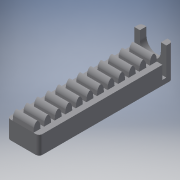
# Autodesk Inventor part: Rack_arms
Saved by Autodesk Inventor 2018 (Build 220112000, 112)
## iProperties
Created: 2017-05-22
Part Number: Rack_arms
Material: Generic
Document SubType Name: Modeling
Designer: nazardio000
Density: 1 g/cm^3
Appearance: Default
Author: nazardio000
Autodesk Inventor part; units mm, degrees
ref_plane "YZ Plane" through (0, 0, 0) normal (1, 0, 0) x (0, 1, 0)
ref_plane "XZ Plane" through (0, 0, 0) normal (0, 1, 0) x (-1, 0, 0)
ref_plane "XY Plane" through (0, 0, 0) normal (0, 0, 1) x (1, 0, 0)
sketch "Sketch2" plane through (0, 0, 0) normal (1, 0, 0) x (0, 1, 0)
  line L0 (-5.5245, 31.75) -> (-5.5245, -31.75)
  line L1 (-5.5245, -31.75) -> (5.5245, -31.75)
  line L2 (5.5245, -31.75) -> (5.5245, 31.75)
  line L3 (5.5245, 31.75) -> (-5.5245, 31.75)
  line L4 (-5.5245, 31.75) -> (5.5245, -31.75) construction
  line L5 (-5.5245, -31.75) -> (5.5245, 31.75) construction
  point P0 (0, 0)
  dimension "d4" = 63.5
  dimension "d5" = 11.049
  constraints: 12 end point, 2 midpoint, 2 parallel, 1 perpendicular, 1 vertical
  measures "d4" distance of L0.start L0.end
  measures "d5" distance of L1.end L0.end
extrude "Extrusion2" add sketch "Sketch2" along normal mid plane 9.779
sketch "Sketch3" plane through (0, 0, 0) normal (1, 0, 0) x (0, 1, 0)
  line L0 (5.5245, -31.75) -> (5.5245, 31.75) projected
  line L1 (5.5245, 31.9532) -> (5.5245, 29.4132)
  line L2 (5.5245, 31.9532) -> (5.5245, 29.4132)
  arc A0 (8.0645, 30.8543) -> (6.7945, 31.629) centre (6.3804, 29.5218) ccw
  line L3 (8.0645, 30.6737) -> (7.6408, 30.6737)
  arc A1 (6.7945, 29.7184) -> (8.0645, 30.4931) centre (6.3804, 31.8256) ccw
  line L4 (8.0645, 30.8543) -> (8.0645, 30.4931)
  line L5 (5.5245, 31.75) -> (5.5245, -31.75)
  arc A2 (8.0642, -1.6042) -> (8.0645, -1.6033) centre (6.6313, -1.0154) ccw
  line L6 (6.7945, 31.629) -> (5.5245, 31.7489)
  line L7 (6.7945, 29.7184) -> (5.5245, 29.5986)
  line L8 (5.5245, 31.7489) -> (6.7945, 31.629)
  line L9 (6.7945, 29.7184) -> (5.5245, 29.5986)
  line L10 (5.5245, 29.5986) -> (5.5245, 31.7489)
  arc A3 (8.0645, 30.8543) -> (6.7945, 31.629) centre (6.3804, 29.5218) ccw
  arc A4 (6.7945, 29.7184) -> (8.0645, 30.4931) centre (6.3804, 31.8256) ccw
  line L11 (8.0645, 30.8543) -> (8.0645, 30.4931)
  line L12 (8.0645, 27.4448) -> (7.6408, 27.4448)
  line L13 (8.0645, 27.6255) -> (8.0645, 27.2642)
  line L14 (8.0645, 27.6255) -> (8.0645, 27.2642)
  arc A5 (6.7945, 26.4895) -> (8.0645, 27.2642) centre (6.3804, 28.5967) ccw
  arc A6 (8.0645, 27.6255) -> (6.7945, 28.4002) centre (6.3804, 26.293) ccw
  arc A7 (6.7945, 26.4895) -> (8.0645, 27.2642) centre (6.3804, 28.5967) ccw
  arc A8 (8.0645, 27.6255) -> (6.7945, 28.4002) centre (6.3804, 26.293) ccw
  line L15 (5.5245, 28.5211) -> (5.5245, -34.9788)
  line L16 (5.5245, 28.7243) -> (5.5245, 26.1843)
  line L17 (6.7945, 26.4895) -> (5.5245, 26.3697)
  line L18 (5.5245, 28.52) -> (6.7945, 28.4002)
  line L19 (6.7945, 26.4895) -> (5.5245, 26.3697)
  line L20 (5.5245, 26.3697) -> (5.5245, 28.52)
  line L21 (5.5245, 28.7243) -> (5.5245, 26.1843)
  line L22 (6.7945, 28.4002) -> (5.5245, 28.52)
  line L23 (8.0645, 24.216) -> (7.6408, 24.216)
  line L24 (8.0645, 24.3966) -> (8.0645, 24.0353)
  line L25 (8.0645, 24.3966) -> (8.0645, 24.0353)
  arc A9 (6.7945, 23.2606) -> (8.0645, 24.0353) centre (6.3804, 25.3678) ccw
  arc A10 (8.0645, 24.3966) -> (6.7945, 25.1713) centre (6.3804, 23.0641) ccw
  arc A11 (6.7945, 23.2606) -> (8.0645, 24.0353) centre (6.3804, 25.3678) ccw
  arc A12 (8.0645, 24.3966) -> (6.7945, 25.1713) centre (6.3804, 23.0641) ccw
  line L26 (5.5245, 25.2923) -> (5.5245, -38.2077)
  line L27 (5.5245, 25.4955) -> (5.5245, 22.9555)
  line L28 (6.7945, 23.2606) -> (5.5245, 23.1408)
  line L29 (5.5245, 25.2911) -> (6.7945, 25.1713)
  line L30 (6.7945, 23.2606) -> (5.5245, 23.1408)
  line L31 (5.5245, 23.1408) -> (5.5245, 25.2911)
  line L32 (5.5245, 25.4955) -> (5.5245, 22.9555)
  line L33 (6.7945, 25.1713) -> (5.5245, 25.2911)
  line L34 (8.0645, 20.9871) -> (7.6408, 20.9871)
  line L35 (8.0645, 21.1677) -> (8.0645, 20.8065)
  line L36 (8.0645, 21.1677) -> (8.0645, 20.8065)
  arc A13 (6.7945, 20.0318) -> (8.0645, 20.8065) centre (6.3804, 22.139) ccw
  arc A14 (8.0645, 21.1677) -> (6.7945, 21.9424) centre (6.3804, 19.8352) ccw
  arc A15 (6.7945, 20.0318) -> (8.0645, 20.8065) centre (6.3804, 22.139) ccw
  arc A16 (8.0645, 21.1677) -> (6.7945, 21.9424) centre (6.3804, 19.8352) ccw
  line L37 (5.5245, 22.0634) -> (5.5245, -41.4366)
  line L38 (5.5245, 22.2666) -> (5.5245, 19.7266)
  line L39 (6.7945, 20.0318) -> (5.5245, 19.9119)
  line L40 (5.5245, 22.0623) -> (6.7945, 21.9424)
  line L41 (6.7945, 20.0318) -> (5.5245, 19.9119)
  line L42 (5.5245, 19.9119) -> (5.5245, 22.0623)
  line L43 (5.5245, 22.2666) -> (5.5245, 19.7266)
  line L44 (6.7945, 21.9424) -> (5.5245, 22.0623)
  line L45 (8.0645, 17.7582) -> (7.6408, 17.7582)
  line L46 (8.0645, 17.9389) -> (8.0645, 17.5776)
  line L47 (8.0645, 17.9389) -> (8.0645, 17.5776)
  arc A17 (6.7945, 16.8029) -> (8.0645, 17.5776) centre (6.3804, 18.9101) ccw
  arc A18 (8.0645, 17.9389) -> (6.7945, 18.7136) centre (6.3804, 16.6064) ccw
  arc A19 (6.7945, 16.8029) -> (8.0645, 17.5776) centre (6.3804, 18.9101) ccw
  arc A20 (8.0645, 17.9389) -> (6.7945, 18.7136) centre (6.3804, 16.6064) ccw
  line L48 (5.5245, 18.8345) -> (5.5245, -44.6655)
  line L49 (5.5245, 19.0377) -> (5.5245, 16.4977)
  line L50 (6.7945, 16.8029) -> (5.5245, 16.6831)
  line L51 (5.5245, 18.8334) -> (6.7945, 18.7136)
  line L52 (6.7945, 16.8029) -> (5.5245, 16.6831)
  line L53 (5.5245, 16.6831) -> (5.5245, 18.8334)
  line L54 (5.5245, 19.0377) -> (5.5245, 16.4977)
  line L55 (6.7945, 18.7136) -> (5.5245, 18.8334)
  line L56 (8.0645, 14.5294) -> (7.6408, 14.5294)
  line L57 (8.0645, 14.71) -> (8.0645, 14.3487)
  line L58 (8.0645, 14.71) -> (8.0645, 14.3487)
  arc A21 (6.7945, 13.574) -> (8.0645, 14.3487) centre (6.3804, 15.6812) ccw
  arc A22 (8.0645, 14.71) -> (6.7945, 15.4847) centre (6.3804, 13.3775) ccw
  arc A23 (6.7945, 13.574) -> (8.0645, 14.3487) centre (6.3804, 15.6812) ccw
  arc A24 (8.0645, 14.71) -> (6.7945, 15.4847) centre (6.3804, 13.3775) ccw
  line L59 (5.5245, 15.6057) -> (5.5245, -47.8943)
  line L60 (5.5245, 15.8089) -> (5.5245, 13.2689)
  line L61 (6.7945, 13.574) -> (5.5245, 13.4542)
  line L62 (5.5245, 15.6045) -> (6.7945, 15.4847)
  line L63 (6.7945, 13.574) -> (5.5245, 13.4542)
  line L64 (5.5245, 13.4542) -> (5.5245, 15.6045)
  line L65 (5.5245, 15.8089) -> (5.5245, 13.2689)
  line L66 (6.7945, 15.4847) -> (5.5245, 15.6045)
  line L67 (8.0645, 11.3005) -> (7.6408, 11.3005)
  line L68 (8.0645, 11.4811) -> (8.0645, 11.1199)
  line L69 (8.0645, 11.4811) -> (8.0645, 11.1199)
  arc A25 (6.7945, 10.3452) -> (8.0645, 11.1199) centre (6.3804, 12.4524) ccw
  arc A26 (8.0645, 11.4811) -> (6.7945, 12.2558) centre (6.3804, 10.1486) ccw
  arc A27 (6.7945, 10.3452) -> (8.0645, 11.1199) centre (6.3804, 12.4524) ccw
  arc A28 (8.0645, 11.4811) -> (6.7945, 12.2558) centre (6.3804, 10.1486) ccw
  line L70 (5.5245, 12.3768) -> (5.5245, -51.1232)
  line L71 (5.5245, 12.58) -> (5.5245, 10.04)
  line L72 (6.7945, 10.3452) -> (5.5245, 10.2253)
  line L73 (5.5245, 12.3756) -> (6.7945, 12.2558)
  line L74 (6.7945, 10.3452) -> (5.5245, 10.2253)
  line L75 (5.5245, 10.2253) -> (5.5245, 12.3756)
  line L76 (5.5245, 12.58) -> (5.5245, 10.04)
  line L77 (6.7945, 12.2558) -> (5.5245, 12.3756)
  line L78 (8.0645, 8.0716) -> (7.6408, 8.0716)
  line L79 (8.0645, 8.2523) -> (8.0645, 7.891)
  line L80 (8.0645, 8.2523) -> (8.0645, 7.891)
  arc A29 (6.7945, 7.1163) -> (8.0645, 7.891) centre (6.3804, 9.2235) ccw
  arc A30 (8.0645, 8.2523) -> (6.7945, 9.027) centre (6.3804, 6.9198) ccw
  arc A31 (6.7945, 7.1163) -> (8.0645, 7.891) centre (6.3804, 9.2235) ccw
  arc A32 (8.0645, 8.2523) -> (6.7945, 9.027) centre (6.3804, 6.9198) ccw
  line L81 (5.5245, 9.1479) -> (5.5245, -54.3521)
  line L82 (5.5245, 9.3511) -> (5.5245, 6.8111)
  line L83 (6.7945, 7.1163) -> (5.5245, 6.9965)
  line L84 (5.5245, 9.1468) -> (6.7945, 9.027)
  line L85 (6.7945, 7.1163) -> (5.5245, 6.9965)
  line L86 (5.5245, 6.9965) -> (5.5245, 9.1468)
  line L87 (5.5245, 9.3511) -> (5.5245, 6.8111)
  line L88 (6.7945, 9.027) -> (5.5245, 9.1468)
  line L89 (8.0645, 4.8428) -> (7.6408, 4.8428)
  line L90 (8.0645, 5.0234) -> (8.0645, 4.6621)
  line L91 (8.0645, 5.0234) -> (8.0645, 4.6621)
  arc A33 (6.7945, 3.8874) -> (8.0645, 4.6621) centre (6.3804, 5.9946) ccw
  arc A34 (8.0645, 5.0234) -> (6.7945, 5.7981) centre (6.3804, 3.6909) ccw
  arc A35 (6.7945, 3.8874) -> (8.0645, 4.6621) centre (6.3804, 5.9946) ccw
  arc A36 (8.0645, 5.0234) -> (6.7945, 5.7981) centre (6.3804, 3.6909) ccw
  line L92 (5.5245, 5.9191) -> (5.5245, -57.5809)
  line L93 (5.5245, 6.1223) -> (5.5245, 3.5823)
  line L94 (6.7945, 3.8874) -> (5.5245, 3.7676)
  line L95 (5.5245, 5.9179) -> (6.7945, 5.7981)
  line L96 (6.7945, 3.8874) -> (5.5245, 3.7676)
  line L97 (5.5245, 3.7676) -> (5.5245, 5.9179)
  line L98 (5.5245, 6.1223) -> (5.5245, 3.5823)
  line L99 (6.7945, 5.7981) -> (5.5245, 5.9179)
  line L100 (8.0645, 1.6139) -> (7.6408, 1.6139)
  line L101 (8.0645, 1.7945) -> (8.0645, 1.4333)
  line L102 (8.0645, 1.7945) -> (8.0645, 1.4333)
  arc A37 (6.7945, 0.6586) -> (8.0645, 1.4333) centre (6.3804, 2.7658) ccw
  arc A38 (8.0645, 1.7945) -> (6.7945, 2.5692) centre (6.3804, 0.462) ccw
  arc A39 (6.7945, 0.6586) -> (8.0645, 1.4333) centre (6.3804, 2.7658) ccw
  arc A40 (8.0645, 1.7945) -> (6.7945, 2.5692) centre (6.3804, 0.462) ccw
  line L103 (5.5245, 2.6902) -> (5.5245, -60.8098)
  line L104 (5.5245, 2.8934) -> (5.5245, 0.3534)
  line L105 (6.7945, 0.6586) -> (5.5245, 0.5387)
  line L106 (5.5245, 2.689) -> (6.7945, 2.5692)
  line L107 (6.7945, 0.6586) -> (5.5245, 0.5387)
  line L108 (5.5245, 0.5387) -> (5.5245, 2.689)
  line L109 (5.5245, 2.8934) -> (5.5245, 0.3534)
  line L110 (6.7945, 2.5692) -> (5.5245, 2.689)
  line L111 (8.0645, -1.615) -> (7.6408, -1.615)
  line L112 (8.0645, -1.4344) -> (8.0645, -1.7956)
  line L113 (8.0645, -1.4344) -> (8.0645, -1.7956)
  arc A41 (6.7945, -2.5703) -> (8.0645, -1.7956) centre (6.3804, -0.4631) ccw
  arc A42 (8.0645, -1.4344) -> (6.7945, -0.6597) centre (6.3804, -2.7668) ccw
  arc A43 (6.7945, -2.5703) -> (8.0645, -1.7956) centre (6.3804, -0.4631) ccw
  arc A44 (8.0645, -1.4344) -> (6.7945, -0.6597) centre (6.3804, -2.7668) ccw
  line L114 (5.5245, -0.5387) -> (5.5245, -64.0387)
  line L115 (5.5245, -0.3355) -> (5.5245, -2.8755)
  line L116 (6.7945, -2.5703) -> (5.5245, -2.6901)
  line L117 (5.5245, -0.5398) -> (6.7945, -0.6597)
  line L118 (6.7945, -2.5703) -> (5.5245, -2.6901)
  line L119 (5.5245, -2.6901) -> (5.5245, -0.5398)
  line L120 (5.5245, -0.3355) -> (5.5245, -2.8755)
  line L121 (6.7945, -0.6597) -> (5.5245, -0.5398)
  line L122 (8.0645, -4.8438) -> (7.6408, -4.8438)
  line L123 (8.0645, -4.6632) -> (8.0645, -5.0245)
  line L124 (8.0645, -4.6632) -> (8.0645, -5.0245)
  arc A45 (6.7945, -5.7992) -> (8.0645, -5.0245) centre (6.3804, -3.692) ccw
  arc A46 (8.0645, -4.6632) -> (6.7945, -3.8885) centre (6.3804, -5.9957) ccw
  arc A47 (6.7945, -5.7992) -> (8.0645, -5.0245) centre (6.3804, -3.692) ccw
  arc A48 (8.0645, -4.6632) -> (6.7945, -3.8885) centre (6.3804, -5.9957) ccw
  line L125 (5.5245, -3.7676) -> (5.5245, -67.2675)
  line L126 (5.5245, -3.5644) -> (5.5245, -6.1044)
  line L127 (6.7945, -5.7992) -> (5.5245, -5.919)
  line L128 (5.5245, -3.7687) -> (6.7945, -3.8885)
  line L129 (6.7945, -5.7992) -> (5.5245, -5.919)
  line L130 (5.5245, -5.919) -> (5.5245, -3.7687)
  line L131 (5.5245, -3.5644) -> (5.5245, -6.1044)
  line L132 (6.7945, -3.8885) -> (5.5245, -3.7687)
  line L133 (8.0645, -8.0727) -> (7.6408, -8.0727)
  line L134 (8.0645, -7.8921) -> (8.0645, -8.2533)
  line L135 (8.0645, -7.8921) -> (8.0645, -8.2533)
  arc A49 (6.7945, -9.028) -> (8.0645, -8.2533) centre (6.3804, -6.9208) ccw
  arc A50 (8.0645, -7.8921) -> (6.7945, -7.1174) centre (6.3804, -9.2246) ccw
  arc A51 (6.7945, -9.028) -> (8.0645, -8.2533) centre (6.3804, -6.9208) ccw
  arc A52 (8.0645, -7.8921) -> (6.7945, -7.1174) centre (6.3804, -9.2246) ccw
  line L136 (5.5245, -6.9964) -> (5.5245, -70.4964)
  line L137 (5.5245, -6.7932) -> (5.5245, -9.3332)
  line L138 (6.7945, -9.028) -> (5.5245, -9.1479)
  line L139 (5.5245, -6.9976) -> (6.7945, -7.1174)
  line L140 (6.7945, -9.028) -> (5.5245, -9.1479)
  line L141 (5.5245, -9.1479) -> (5.5245, -6.9976)
  line L142 (5.5245, -6.7932) -> (5.5245, -9.3332)
  line L143 (6.7945, -7.1174) -> (5.5245, -6.9976)
  line L144 (8.0645, -11.3016) -> (7.6408, -11.3016)
  line L145 (8.0645, -11.121) -> (8.0645, -11.4822)
  line L146 (8.0645, -11.121) -> (8.0645, -11.4822)
  arc A53 (6.7945, -12.2569) -> (8.0645, -11.4822) centre (6.3804, -10.1497) ccw
  arc A54 (8.0645, -11.121) -> (6.7945, -10.3463) centre (6.3804, -12.4535) ccw
  arc A55 (6.7945, -12.2569) -> (8.0645, -11.4822) centre (6.3804, -10.1497) ccw
  arc A56 (8.0645, -11.121) -> (6.7945, -10.3463) centre (6.3804, -12.4535) ccw
  line L147 (5.5245, -10.2253) -> (5.5245, -73.7253)
  line L148 (5.5245, -10.0221) -> (5.5245, -12.5621)
  line L149 (6.7945, -12.2569) -> (5.5245, -12.3767)
  line L150 (5.5245, -10.2264) -> (6.7945, -10.3463)
  line L151 (6.7945, -12.2569) -> (5.5245, -12.3767)
  line L152 (5.5245, -12.3767) -> (5.5245, -10.2264)
  line L153 (5.5245, -10.0221) -> (5.5245, -12.5621)
  line L154 (6.7945, -10.3463) -> (5.5245, -10.2264)
  line L155 (8.0645, -14.5305) -> (7.6408, -14.5305)
  line L156 (8.0645, -14.3498) -> (8.0645, -14.7111)
  line L157 (8.0645, -14.3498) -> (8.0645, -14.7111)
  arc A57 (6.7945, -15.4858) -> (8.0645, -14.7111) centre (6.3804, -13.3786) ccw
  arc A58 (8.0645, -14.3498) -> (6.7945, -13.5751) centre (6.3804, -15.6823) ccw
  arc A59 (6.7945, -15.4858) -> (8.0645, -14.7111) centre (6.3804, -13.3786) ccw
  arc A60 (8.0645, -14.3498) -> (6.7945, -13.5751) centre (6.3804, -15.6823) ccw
  line L158 (5.5245, -13.4542) -> (5.5245, -76.9541)
  line L159 (5.5245, -13.251) -> (5.5245, -15.791)
  line L160 (6.7945, -15.4858) -> (5.5245, -15.6056)
  line L161 (5.5245, -13.4553) -> (6.7945, -13.5751)
  line L162 (6.7945, -15.4858) -> (5.5245, -15.6056)
  line L163 (5.5245, -15.6056) -> (5.5245, -13.4553)
  line L164 (5.5245, -13.251) -> (5.5245, -15.791)
  line L165 (6.7945, -13.5751) -> (5.5245, -13.4553)
  line L166 (8.0645, -17.7593) -> (7.6408, -17.7593)
  line L167 (8.0645, -17.5787) -> (8.0645, -17.9399)
  line L168 (8.0645, -17.5787) -> (8.0645, -17.9399)
  arc A61 (6.7945, -18.7146) -> (8.0645, -17.9399) centre (6.3804, -16.6075) ccw
  arc A62 (8.0645, -17.5787) -> (6.7945, -16.804) centre (6.3804, -18.9112) ccw
  arc A63 (6.7945, -18.7146) -> (8.0645, -17.9399) centre (6.3804, -16.6075) ccw
  arc A64 (8.0645, -17.5787) -> (6.7945, -16.804) centre (6.3804, -18.9112) ccw
  line L169 (5.5245, -16.683) -> (5.5245, -80.183)
  line L170 (5.5245, -16.4798) -> (5.5245, -19.0198)
  line L171 (6.7945, -18.7146) -> (5.5245, -18.8345)
  line L172 (5.5245, -16.6842) -> (6.7945, -16.804)
  line L173 (6.7945, -18.7146) -> (5.5245, -18.8345)
  line L174 (5.5245, -18.8345) -> (5.5245, -16.6842)
  line L175 (5.5245, -16.4798) -> (5.5245, -19.0198)
  line L176 (6.7945, -16.804) -> (5.5245, -16.6842)
  line L177 (8.0645, -20.9882) -> (7.6408, -20.9882)
  line L178 (8.0645, -20.8076) -> (8.0645, -21.1688)
  line L179 (8.0645, -20.8076) -> (8.0645, -21.1688)
  arc A65 (6.7945, -21.9435) -> (8.0645, -21.1688) centre (6.3804, -19.8363) ccw
  arc A66 (8.0645, -20.8076) -> (6.7945, -20.0329) centre (6.3804, -22.1401) ccw
  arc A67 (6.7945, -21.9435) -> (8.0645, -21.1688) centre (6.3804, -19.8363) ccw
  arc A68 (8.0645, -20.8076) -> (6.7945, -20.0329) centre (6.3804, -22.1401) ccw
  line L180 (5.5245, -19.9119) -> (5.5245, -83.4119)
  line L181 (5.5245, -19.7087) -> (5.5245, -22.2487)
  line L182 (6.7945, -21.9435) -> (5.5245, -22.0633)
  line L183 (5.5245, -19.913) -> (6.7945, -20.0329)
  line L184 (6.7945, -21.9435) -> (5.5245, -22.0633)
  line L185 (5.5245, -22.0633) -> (5.5245, -19.913)
  line L186 (5.5245, -19.7087) -> (5.5245, -22.2487)
  line L187 (6.7945, -20.0329) -> (5.5245, -19.913)
  line L188 (8.0645, -24.2171) -> (7.6408, -24.2171)
  line L189 (8.0645, -24.0364) -> (8.0645, -24.3977)
  line L190 (8.0645, -24.0364) -> (8.0645, -24.3977)
  arc A69 (6.7945, -25.1724) -> (8.0645, -24.3977) centre (6.3804, -23.0652) ccw
  arc A70 (8.0645, -24.0364) -> (6.7945, -23.2617) centre (6.3804, -25.3689) ccw
  arc A71 (6.7945, -25.1724) -> (8.0645, -24.3977) centre (6.3804, -23.0652) ccw
  arc A72 (8.0645, -24.0364) -> (6.7945, -23.2617) centre (6.3804, -25.3689) ccw
  line L191 (5.5245, -23.1408) -> (5.5245, -86.6407)
  line L192 (5.5245, -22.9376) -> (5.5245, -25.4776)
  line L193 (6.7945, -25.1724) -> (5.5245, -25.2922)
  line L194 (5.5245, -23.1419) -> (6.7945, -23.2617)
  line L195 (6.7945, -25.1724) -> (5.5245, -25.2922)
  line L196 (5.5245, -25.2922) -> (5.5245, -23.1419)
  line L197 (5.5245, -22.9376) -> (5.5245, -25.4776)
  line L198 (6.7945, -23.2617) -> (5.5245, -23.1419)
  line L199 (8.0645, -27.4459) -> (7.6408, -27.4459)
  line L200 (8.0645, -27.2653) -> (8.0645, -27.6266)
  line L201 (8.0645, -27.2653) -> (8.0645, -27.6266)
  arc A73 (6.7945, -28.4013) -> (8.0645, -27.6266) centre (6.3804, -26.2941) ccw
  arc A74 (8.0645, -27.2653) -> (6.7945, -26.4906) centre (6.3804, -28.5978) ccw
  arc A75 (6.7945, -28.4013) -> (8.0645, -27.6266) centre (6.3804, -26.2941) ccw
  arc A76 (8.0645, -27.2653) -> (6.7945, -26.4906) centre (6.3804, -28.5978) ccw
  line L202 (5.5245, -26.3696) -> (5.5245, -89.8696)
  line L203 (5.5245, -26.1664) -> (5.5245, -28.7064)
  line L204 (6.7945, -28.4013) -> (5.5245, -28.5211)
  line L205 (5.5245, -26.3708) -> (6.7945, -26.4906)
  line L206 (6.7945, -28.4013) -> (5.5245, -28.5211)
  line L207 (5.5245, -28.5211) -> (5.5245, -26.3708)
  line L208 (5.5245, -26.1664) -> (5.5245, -28.7064)
  line L209 (6.7945, -26.4906) -> (5.5245, -26.3708)
  line L210 (8.0645, -30.6748) -> (7.6408, -30.6748)
  line L211 (8.0645, -30.4942) -> (8.0645, -30.8554)
  line L212 (8.0645, -30.4942) -> (8.0645, -30.8554)
  arc A77 (6.7945, -31.6301) -> (8.0645, -30.8554) centre (6.3804, -29.5229) ccw
  arc A78 (8.0645, -30.4942) -> (6.7945, -29.7195) centre (6.3804, -31.8267) ccw
  arc A79 (6.7945, -31.6301) -> (8.0645, -30.8554) centre (6.3804, -29.5229) ccw
  arc A80 (8.0645, -30.4942) -> (6.7945, -29.7195) centre (6.3804, -31.8267) ccw
  line L213 (5.5245, -29.5985) -> (5.5245, -93.0985)
  line L214 (5.5245, -29.3953) -> (5.5245, -31.9353)
  line L215 (6.7945, -31.6301) -> (5.5245, -31.7499)
  line L216 (5.5245, -29.5996) -> (6.7945, -29.7195)
  line L217 (6.7945, -31.6301) -> (5.5245, -31.7499)
  line L218 (5.5245, -31.7499) -> (5.5245, -29.5996)
  line L219 (5.5245, -29.3953) -> (5.5245, -31.9353)
  line L220 (6.7945, -29.7195) -> (5.5245, -29.5996)
  point P0 (0, 0)
  point P1 (6.7953, 29.7185)
  point P2 (6.7953, 26.4897)
  point P3 (6.7953, 23.2608)
  point P4 (6.7953, 20.0319)
  point P5 (6.7953, 16.8031)
  point P6 (6.7953, 13.5742)
  point P7 (6.7953, 10.3453)
  point P8 (6.7953, 7.1164)
  point P9 (6.7953, 3.8876)
  point P10 (6.7953, 0.6587)
  point P11 (6.7953, -2.5702)
  point P12 (6.7953, -5.799)
  point P13 (6.7953, -9.0279)
  point P14 (6.7953, -12.2568)
  point P15 (6.7953, -15.4856)
  point P16 (6.7953, -18.7145)
  point P17 (6.7953, -21.9434)
  point P18 (6.7953, -25.1722)
  point P19 (6.7953, -28.4011)
  point P20 (6.7953, -31.63)
  dimension "d9" = 2.3368
  dimension "d63" = 84.61
  dimension "d64" = 84.61
  dimension "d74" = 3.2289
  constraints: 402 end point, 182 point on circle, 81 centre point, 20 coincident, 5 collinear, 3 symmetric about line, 2 concentric, 2 vertical, 1 horizontal, 628 other
  measures "d9" distance of L0.end L1.end
  measures "d63" angle of L0 L6
  measures "d64" angle of L0 L7
  measures "d74" distance of L1.end L16.end
sketch "Sketch5" plane through (-4.8895, -5.5245, 31.75) normal (0, -1, 0) x (1, 0, 0)
  line L0 (9.779, 0) -> (9.779, -63.5) projected
  line L1 (9.779, 0) -> (0, 0) projected
  line L2 (0, -63.5) -> (0, 0) projected
  line L3 (0, -63.5) -> (0, 0) projected
  line L4 (0, -63.5) -> (9.779, -63.5) projected
  line L5 (0, -63.5) -> (9.779, -63.5) projected
  line L6 (9.779, 0) -> (9.779, -63.5) projected
  line L7 (9.779, 0) -> (0, 0) projected
  line L8 (0, -63.5) -> (0, 0) projected
  line L9 (9.779, 0) -> (9.779, -63.5) projected
  line L10 (9.779, 0) -> (0, 0) projected
  line L11 (0, -63.5) -> (9.779, -63.5) projected
  point P0 (4.8895, -31.75)
extrude "Extrusion6" add sketch "Sketch5" along normal blind 2.54
sketch "Sketch6" plane through (4.8895, 0, 0) normal (1, 0, 0) x (0, 0, -1)
  line L0 (31.75, 5.5245) -> (31.75, -8.0645) projected
  line L1 (27.9384, 4.6355) -> (31.75, 4.6355)
  line L2 (31.75, 4.6355) -> (31.75, 2.0955)
  line L3 (31.75, 2.0955) -> (27.9384, 2.0955)
  line L4 (27.9384, 2.0955) -> (27.9384, 4.6355)
  point P0 (0, 0)
  dimension "d60" = 2.54
  constraints: 8 end point, 2 parallel, 1 horizontal, 1 perpendicular, 1 point on line
  measures "d60" distance of L3.end L1.start
extrude "Extrusion7" add sketch "Sketch6" against normal blind 9.779
extrude "Extrusion8" add sketch "Sketch3" along normal mid plane 6.35 contours L0 L6 A0 L4 A1 L7 | L0 L18 A6 L13 A5 L17 | L0 L29 A10 L24 A9 L28 | L0 L40 A14 L35 A13 L39 | L0 L51 A18 L46 A17 L50 | L0 L62 A22 L57 A21 L61 | L0 L73 A26 L68 A25 L72 | L0 L84 A30 L79 A29 L83 | L0 L95 A34 L90 A33 L94 | L0 L106 A38 L101 A37 L105 | L0 A2 A41 L116 | L0 L128 A46 L123 A45 L127 | L0 L139 A50 L134 A49 L138 | L0 L150 A54 L145 A53 L149 | L0 L161 A58 L156 A57 L160 | L0 L172 A62 L167 A61 L171 | L0 L183 A66 L178 A65 L182 | L0 L194 A70 L189 A69 L193 | L0 L205 A74 L200 A73 L204 | L0 L216 A78 L211 A77 L215 | L0 L117 A42 L112 A2 A41 | A2 L111 L112 A41 | L112 L111 A2
sketch "Sketch7" plane through (4.8895, 0, 0) normal (1, 0, 0) x (0, 0, -1)
  line L0 (29.2084, 2.0955) -> (31.75, 2.0955) projected
  line L1 (27.9384, 2.0955) -> (27.9384, -8.0645) projected
  line L2 (29.2084, 2.0955) -> (27.9384, 2.0955)
  line L3 (27.9384, 2.0955) -> (27.9384, -8.0645)
  line L4 (27.9384, -8.0645) -> (29.2084, -8.0645)
  line L5 (29.2084, -8.0645) -> (29.2084, 2.0955)
  line L6 (27.9384, -8.0645) -> (26.6684, -8.0645)
  line L7 (26.6684, -8.0645) -> (26.6684, 2.0955)
  line L8 (26.6684, 2.0955) -> (27.9384, 2.0955)
  line L9 (27.9384, 2.0955) -> (27.9384, -8.0645)
  point P0 (0, 0)
  dimension "d81" = 1.27
  constraints: 16 end point, 4 parallel, 2 horizontal, 2 perpendicular
  measures "d81" distance of L7.end L8.end
extrude "Extrusion9" add sketch "Sketch7" against normal blind 9.779 contours L2 L5 L4 L1
sketch "Sketch8" plane through (4.8895, 0, 0) normal (1, 0, 0) x (0, 0, -1)
  line L0 (31.75, -8.0645) -> (29.2084, -8.0645) projected
  line L1 (31.75, -8.0645) -> (27.94, -8.0645)
  line L2 (-31.75, -8.0645) -> (31.75, -8.0645) projected
  line L3 (27.94, -8.0645) -> (26.67, -8.0645)
  line L4 (27.94, -8.0645) -> (27.94, 2.0955)
  line L5 (27.94, 2.0955) -> (26.67, 2.0955)
  line L6 (26.67, 2.0955) -> (26.67, -8.0645)
  point P0 (0, 0)
  dimension "d84" = 3.81
  dimension "d85" = 1.27
  dimension "d86" = 10.16
  constraints: 10 end point, 2 perpendicular, 2 point on line, 1 vertical
  measures "d84" distance of L0.start L1.end
  measures "d85" distance of L1.end L3.end
  measures "d86" distance of L1.end L4.end
extrude "Extrusion10" cut sketch "Sketch8" against normal blind 9.779
sketch "Sketch9" plane through (4.8895, -8.0645, -27.94) normal (0, 0, 1) x (1, 0, 0)
  line L0 (-6.7945, 0) -> (-6.7945, 10.16) projected
  line L1 (-2.9845, 10.16) -> (-6.7945, 10.16) projected
  line L2 (-2.9845, 10.16) -> (-2.9845, 0) projected
  line L3 (-2.9845, 0) -> (-6.7945, 0) projected
  point P0 (-4.8895, 8.0645)
extrude "Extrusion11" cut sketch "Sketch9" against normal blind 9.779
sketch "Sketch10" plane through (4.8895, 0, 0) normal (1, 0, 0) x (0, 0, -1)
  line L0 (31.75, 2.0955) -> (31.75, -8.0645) projected
  line L1 (31.75, -8.0645) -> (-31.75, -8.0645)
  line L2 (31.7499, 5.5245) -> (29.5996, 5.5245) projected
  line L3 (-31.7501, 4.5245) -> (31.7499, 4.5245)
  line L4 (31.75, 5.5245) -> (31.75, -8.0645) projected
  line L5 (-31.7501, 4.5245) -> (31.75, 4.5245)
  line L6 (31.75, 4.5245) -> (31.75, -8.0645)
  line L7 (31.75, -8.0645) -> (-31.7501, -8.0645)
  line L8 (-31.7501, -8.0645) -> (-31.7501, 4.5245)
  point P0 (0, 0)
  dimension "d93" = 63.5
  constraints: 12 end point, 2 parallel, 1 horizontal, 1 perpendicular
  measures "d93" distance of L3.end L3.start
extrude "Extrusion12" cut sketch "Sketch10" against normal blind 25.4
sketch "Sketch11" plane through (4.8895, 4.5245, -31.75) normal (0, -1, 0) x (1, 0, 0)
  line L0 (-9.779, 63.5) -> (0, 63.5) projected
  line L1 (-9.779, 0) -> (-9.779, 63.5) projected
  line L2 (0, 0) -> (-9.779, 0) projected
  line L3 (0, 63.5) -> (0, 0) projected
  point P0 (-4.8895, 31.75)
extrude "Extrusion13" add sketch "Sketch11" along normal blind 3.5
sketch "Sketch12" plane through (4.8895, 1.0245, -31.75) normal (0, -1, 0) x (1, 0, 0)
  line L0 (0, 63.5) -> (-9.779, 63.5) projected
  line L1 (-9.779, 63.5) -> (-9.779, 0) projected
  line L2 (-9.779, 0) -> (0, 0) projected
  line L3 (0, 0) -> (0, 63.5) projected
  line L4 (0, 63.5) -> (-9.779, 63.5)
  line L5 (-9.779, 63.5) -> (-9.779, 69.85)
  line L6 (-9.779, 69.85) -> (0, 69.85)
  line L7 (0, 69.85) -> (0, 63.5)
  line L8 (0, 0) -> (0, 63.5) projected
  line L9 (0, 0) -> (-9.779, 0)
  line L10 (-9.779, 0) -> (-9.779, -6.35)
  line L11 (-9.779, -6.35) -> (0, -6.35)
  line L12 (0, -6.35) -> (0, 0)
  point P0 (-4.8895, 31.75)
  dimension "d97" = 6.35
  dimension "d98" = 6.35
  constraints: 16 end point, 4 parallel, 2 horizontal, 2 perpendicular
  measures "d97" distance of L4.end L5.end
  measures "d98" distance of L9.end L10.end
extrude "Extrusion14" add sketch "Sketch12" along normal blind 1
sketch "Sketch13" plane through (4.8895, 1.0245, -31.75) normal (0, 1, 0) x (1, 0, 0)
  line L0 (0, -69.85) -> (-9.779, -69.85) projected
  line L1 (0, -63.5) -> (0, -69.85) projected
  line L2 (-9.779, 6.35) -> (0, 6.35) projected
  line L3 (0, 6.35) -> (0, 0) projected
  circle A0 centre (-4.8895, 3.175) radius 1.25
  circle A1 centre (-4.8895, -66.675) radius 1.25
  point P0 (-4.8895, -31.75)
  point P1 (-4.8895, -69.85)
  point P2 (0, -66.675)
  point P3 (-4.8895, 6.35)
  point P4 (0, 3.175)
  dimension "d101" = 2.5
  dimension "d102" = 2.5
  constraints: 4 midpoint, 2 centre point
  measures "d101" diameter of A0
  measures "d102" diameter of A1
extrude "Extrusion15" cut sketch "Sketch13" against normal blind 1
sketch "Sketch14" plane through (-3.8895, 5.5245, 31.75) normal (0, 1, 0) x (1, 0, 0)
  line L0 (-2.3413, 37.669) -> (16.7384, 37.669)
  line L1 (16.7384, 37.669) -> (16.7384, 74.3036)
  line L2 (16.7384, 74.3036) -> (-2.3413, 74.3036)
  line L3 (-2.3413, 74.3036) -> (-2.3413, 37.669)
  line L4 (8.779, 0) -> (-1, 0) projected
  line L5 (-1, 0) -> (12.5409, 0)
  line L6 (12.5409, 0) -> (12.5409, -8.7328)
  line L7 (12.5409, -8.7328) -> (-1, -8.7328)
  line L8 (-1, -8.7328) -> (-1, 0)
  point P0 (3.8895, 31.75)
  constraints: 16 end point, 4 parallel, 2 horizontal, 2 perpendicular
extrude "Extrusion16" cut sketch "Sketch14" along normal mid plane 25.4
sketch "Sketch15" plane through (-3.175, 5.5245, -5.919) normal (0, 0, -1) x (-1, 0, 0)
  line L0 (-8.0645, -5.5) -> (-8.0645, -4.5) projected
  line L1 (1.7145, 0) -> (1.7145, -5.5) projected
  line L2 (-8.0645, -5.5) -> (1.7145, -5.5)
  line L3 (1.7145, -5.5) -> (1.7145, -4)
  line L4 (1.7145, -4) -> (-8.0645, -4)
  line L5 (-8.0645, -4) -> (-8.0645, -5.5)
  point P0 (-3.175, -5.5245)
  point P1 (1.7145, -1)
  point P2 (1.7145, -4.5)
  dimension "d108" = 1.5
  constraints: 8 end point, 2 parallel, 1 horizontal, 1 perpendicular, 1 point on line
  measures "d108" distance between parallel lines of L2 L4
extrude "Extrusion17" add sketch "Sketch15" along normal blind 1.2
sketch "Sketch16" plane through (-3.175, 5.5245, -7.119) normal (0, 0, -1) x (-1, 0, 0)
  line L0 (-8.0645, -5.5) -> (-8.0645, -4.5) projected
  line L1 (-8.0645, -5.5) -> (-5.075, -5.5)
  line L2 (-7.0645, -5.5) -> (0.7145, -5.5) projected
  line L3 (1.7145, -5.5) -> (0.7145, -5.5) projected
  line L4 (1.7145, -5.5) -> (-1.275, -5.5)
  line L5 (-8.0645, -5.5) -> (1.7145, -5.5) projected
  line L6 (-8.0645, -5.5) -> (-5.075, -5.5)
  line L7 (-5.075, -5.5) -> (-5.075, 4.5)
  line L8 (-5.075, 4.5) -> (-8.0645, 4.5)
  line L9 (-8.0645, 4.5) -> (-8.0645, -5.5)
  line L10 (-1.275, -5.5) -> (1.7145, -5.5)
  line L11 (1.7145, -5.5) -> (1.7145, 4.5)
  line L12 (1.7145, 4.5) -> (-1.275, 4.5)
  line L13 (-1.275, 4.5) -> (-1.275, -5.5)
  circle A0 centre (-3.175, 0.85) radius 1.9 projected
  line L14 (-5.075, -5.5) -> (-1.275, -5.5)
  circle A1 centre (-3.175, 0.85) radius 1.9
  line L15 (-5.075, 0.85) -> (-5.075, -5.5)
  line L16 (-1.275, 0.85) -> (-1.275, -5.5)
  point P0 (-3.175, -5.5245)
  dimension "d111" = 2.9895
  dimension "d112" = 2.9895
  dimension "d113" = 10
  dimension "d114" = 10
  constraints: 26 end point, 4 collinear, 4 parallel, 3 point on line, 2 horizontal, 2 perpendicular, 2 point on circle, 2 tangent, 1 centre point, 1 coincident
  measures "d111" distance of L0.start L1.end
  measures "d112" distance of L3.start L4.end
  measures "d113" distance of L8.end L0.start
  measures "d114" distance of L10.end L11.end
extrude "Extrusion18" add sketch "Sketch16" along normal blind 2 contours L0 L9 L8 L7 L1 | L7 A0 L13 L2 | L13 L12 L11 L3 L2
sketch "Sketch17" plane through (-3.175, 5.5245, -9.119) normal (0, 0, -1) x (-1, 0, 0)
  circle A0 centre (-3.175, 2) radius 3.2 projected
  line L0 (-6.375, 2) -> (-6.375, 4.5)
  line L1 (-5.075, 4.5) -> (-8.0645, 4.5) projected
  line L2 (0.025, 2) -> (0.025, 4.5)
  line L3 (0.025, 4.5) -> (-6.375, 4.5)
  circle A1 centre (-3.175, 2) radius 3.2
  line L4 (-6.375, 2) -> (0.025, 2)
  line L5 (0.025, 2) -> (0.025, 4.5)
  line L6 (0.025, 4.5) -> (-6.375, 4.5)
  line L7 (-6.375, 4.5) -> (-6.375, 2)
  point P0 (-3.175, -5.5245)
  constraints: 14 end point, 3 parallel, 2 perpendicular, 2 point on circle, 1 coincident, 1 horizontal, 1 horizontal alignment, 1 point on line, 1 tangent, 1 vertical, 2 other
extrude "Extrusion19" cut sketch "Sketch17" against normal up to surface (2 mm away)
fillet "Fillet2" radius 1 4 edges at (-4.8895, 2.7745, 31.75) (4.8895, 2.7745, 31.75) (-4.8895, 5.0245, -9.119) (4.8895, 5.0245, -9.119)
body "Solid2"
